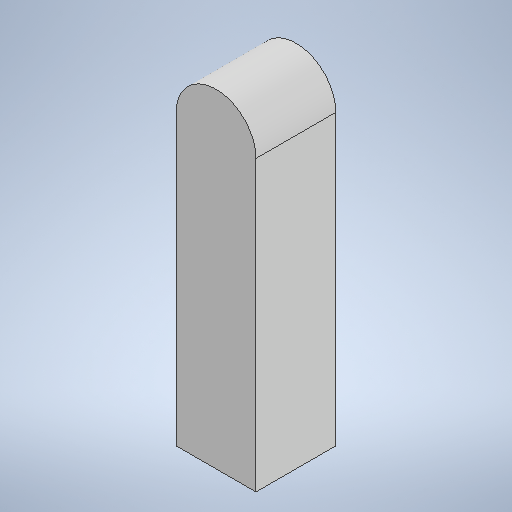
# Autodesk Inventor part: Vane
Saved by Autodesk Inventor 2026.1 (Build 301233020, 233B)
## iProperties
Created: 2025-10-20
Part Number: Vane
Material: Generic
Document SubType Name: Modeling
Designer: yo
Density: 1 g/cm^3
Appearance: Default
Author: yo
Autodesk Inventor part; units mm, degrees
ref_plane "YZ Plane" through (0, 0, 0) normal (1, 0, 0) x (0, 1, 0)
ref_plane "XZ Plane" through (0, 0, 0) normal (0, 1, 0) x (-1, 0, 0)
ref_plane "XY Plane" through (0, 0, 0) normal (0, 0, 1) x (1, 0, 0)
sketch "Sketch1" plane through (0, 0, 0) normal (0, 0, 1) x (1, 0, 0)
  line L0 (-1.3, 5.35) -> (0, 5.35) construction
  line L1 (1.3, 5.35) -> (1.3, 4.05) construction
  line L2 (1.3, -5.35) -> (-1.3, -5.35)
  line L3 (-1.3, -5.35) -> (-1.3, 4.05)
  arc A0 (1.3, 4.05) -> (-1.3, 4.05) centre (0, 4.05) ccw
  line L4 (-1.3, 4.05) -> (-1.3, 5.35) construction
  line L5 (0, 5.35) -> (1.3, 5.35) construction
  line L6 (1.3, 4.05) -> (1.3, -5.35)
  line L7 (0, 5.35) -> (0, -5.35) construction
  point P0 (0, 0)
  point P1 (0, 0)
  dimension "d0" = 10.7
  dimension "d1" = 2.6
  dimension "d3" = 1.3
  constraints: 16 end point, 6 parallel, 5 perpendicular, 3 point on circle, 2 horizontal, 2 midpoint, 2 tangent, 1 centre point, 1 coincident, 1 horizontal alignment, 1 vertical alignment
  measures "d0" distance of L1.start L2.start
  measures "d1" distance of L2.start L2.end
  measures "d3" radius of A0
extrude "Extrusion1" add sketch "Sketch1" along normal blind 2.6
equation "\"d3\" = 0.5 * d1"
body "Solid1"
